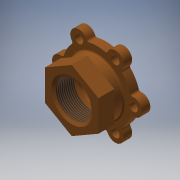
# Autodesk Inventor part: Body Cap
Saved by Autodesk Inventor 2018 (Build 220112000, 112)
## iProperties
Shininess: 64.0
Length Units: 11269
Angle Units: 11279
Time Units: 11290
Mass Units: 11283
Length Display Precision: 3
Angle Display Precision: 2
Created: 2002-03-21
Part Number: Body Cap
Document SubType Name: Modeling
Designer: Default
Material: Bronze, Soft Tin
Density: 8.874 g/cm^3
Appearance: Bronze - Satin
Density: 0.0
Volumn: 0.0
Area: 0.0
PropertySet Name: Model Information
Control State: 0
Master: False
Checked Out: False
Author: Default
Autodesk Inventor part; units mm, degrees
ref_plane "YZ Plane" through (0, 0, 0) normal (1, 0, 0) x (0, 1, 0)
ref_plane "XZ Plane" through (0, 0, 0) normal (0, 1, 0) x (-1, 0, 0)
ref_plane "XY Plane" through (0, 0, 0) normal (0, 0, 1) x (1, 0, 0)
sketch "Sketch1" plane through (0, 0, 0) normal (0, 0, 1) x (1, 0, 0)
  line L0 (-3.9, 0) -> (50.7, 0) projected
  line L1 (0, -3.9) -> (0, 50.7) projected
  line L2 (28.5, 0) -> (28.5, 27)
  line L3 (28.5, 27) -> (37, 27)
  line L4 (37, 27) -> (37, 36)
  line L5 (37, 36) -> (33.5, 36)
  line L6 (33.5, 36) -> (33.5, 33)
  line L7 (33.5, 33) -> (28.5, 33)
  line L8 (28.5, 33) -> (28.5, 39)
  line L9 (28.5, 39) -> (25.5, 39)
  line L10 (25.5, 39) -> (25.5, 29)
  line L11 (25.5, 29) -> (20, 29)
  line L12 (20, 29) -> (20, 26)
  line L13 (20, 26) -> (16, 26)
  line L14 (16, 26) -> (16, 23)
  line L15 (16, 23) -> (19, 21)
  line L16 (19, 21) -> (19, 2)
  line L17 (19, 2) -> (22, 0)
  line L18 (22, 0) -> (28.5, 0)
  dimension "d0" = 3
  dimension "d1" = 32
  dimension "d2" = 38
  dimension "d3" = 57
  dimension "d4" = 40
  dimension "d5" = 51
  dimension "d6" = 57
  dimension "d7" = 74
  dimension "d8" = 5
  dimension "d9" = 2
  dimension "d10" = 21
  dimension "d11" = 23
  dimension "d12" = 26
  dimension "d13" = 29
  dimension "d14" = 27
  dimension "d15" = 33
  dimension "d16" = 36
  dimension "d17" = 39
  constraints: 34 end point, 10 parallel, 4 perpendicular, 2 point on line, 1 collinear
  measures "d0" distance from line of L17.end L16
  measures "d1" diameter of L14 L1
  measures "d2" diameter of L16 L1
  measures "d3" diameter of L2 L1
  measures "d4" diameter of L12 L1
  measures "d5" diameter of L10 L1
  measures "d6" diameter of L8 L1
  measures "d7" diameter of L4 L1
  measures "d8" distance between parallel lines of L6 L8
  measures "d9" distance from line of L16.end L18
  measures "d10" distance from line of L15.end L18
  measures "d11" distance from line of L18 L14.end
  measures "d12" distance between parallel lines of L18 L13
  measures "d13" distance between parallel lines of L18 L11
  measures "d14" distance between parallel lines of L18 L3
  measures "d15" distance between parallel lines of L18 L7
  measures "d16" distance between parallel lines of L18 L5
  measures "d17" distance between parallel lines of L18 L9
revolve "Revolution1" add sketch "Sketch1" angle 360 about axis through (0, -10, 0) along (0, 1, 0)
fillet "Fillet1" radius 2 1 edges at (-28.5, 27, 0)
sketch "Sketch2" plane through (0, 0, 0) normal (0, -1, 0) x (1, 0, 0)
  circle A0 centre (0, 0) radius 28.5 projected
  line L0 (-44.4, 0) -> (59.2, 0) projected
  line L1 (0, -44.4) -> (0, 59.2) projected
  line L2 (0, 32.909) -> (28.5, 16.4545)
  line L3 (28.5, 16.4545) -> (28.5, -16.4545)
  line L4 (28.5, -16.4545) -> (0, -32.909)
  line L5 (0, -32.909) -> (-28.5, -16.4545)
  line L6 (-28.5, -16.4545) -> (-28.5, 16.4545)
  line L7 (-28.5, 16.4545) -> (0, 32.909)
  constraints: 12 end point, 1 coincident, 1 point on line, 1 tangent, 11 other
extrude "Extrusion1" add sketch "Sketch2" against normal blind 17 contours L3 L4 A0 | A0 L2 L3 | A0 L1 L2 | L4 L1 A0 | A0 L7 L1 | L1 L5 A0 | L6 L7 A0 | A0 L5 L6
thread "Thread1" size "M39x2" class "6H" standard "ANSI Metric M Profile" full length
sketch "Sketch3" plane through (0, 36, 0) normal (0, 1, 0) x (1, 0, 0)
  circle A0 centre (0, 0) radius 37 projected
  line L0 (-59.2, 0) -> (44.4, 0) projected
  line L1 (0, 44.4) -> (0, -59.2) projected
  line L2 (35.8887, 9) -> (39, 9)
  arc A1 (39, -9) -> (39, 9) centre (39, 0) ccw
  line L3 (39, -9) -> (35.8887, -9)
  dimension "d24" = 9
  dimension "d25" = 78
  constraints: 4 end point, 4 point on circle, 2 tangent, 1 centre point, 1 parallel, 1 perpendicular, 1 other
  measures "d24" radius of A1
  measures "d25" diameter of A1.centre L1
extrude "Extrusion2" add sketch "Sketch3" against normal blind 9 contours A0 L2 A1 L3
fillet "Fillet2" radius 2 2 edges at (35.8887, 31.5, 9) (35.8887, 31.5, -9)
sketch "Sketch4" plane through (39, 36, 0) normal (0, 1, 0) x (1, 0, 0)
  arc A0 (0, -9) -> (0, 9) centre (0, 0) ccw projected
  constraints: 1 coincident
hole "Hole1" at (39, 36, 0) direction (0, -1, 0) diameter 9 end through all
pattern_circular "Circular Pattern1" count 6 over 360 about axis through (0, 11.5, 0) along (0, -1, 0) of "Extrusion2", "Fillet2", "Hole1"
body "Solid1"
